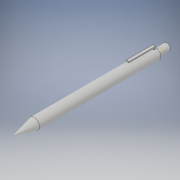
# Autodesk Inventor part: Pen
Saved by Autodesk Inventor 2017 (Build 210142000, 142)
## iProperties
Created: 2018-03-21
Part Number: Pen
Material: Generic
Document SubType Name: Modeling
Designer: landontracy
Density: 1 g/cm^3
Appearance: Default
Author: landontracy
Autodesk Inventor part; units mm, degrees
ref_plane "YZ Plane" through (0, 0, 0) normal (1, 0, 0) x (0, 1, 0)
sketch "Sketch1" plane through (0, 0, 0) normal (0, 0, 1) x (1, 0, 0)
  circle A0 centre (-3.4636, -0.3407) radius 4.445
  point P0 (0, 0)
  dimension "d0" = 8.89
  constraints: 1 centre point
  measures "d0" diameter of A0
extrude "Pen body" add sketch "Sketch1" along normal blind 101.6
ref_plane "Tip Plane" through (-3.4636, -0.3407, 119.38) normal (0, 0, 1) x (1, 0, 0)
sketch "Sketch2" plane through (-3.4636, -0.3407, 119.38) normal (0, 0, 1) x (1, 0, 0)
  circle A0 centre (0, 0) radius 0.0254
  point P0 (3.4636, 0.3407)
  dimension "d4" = 0.0508
  constraints: 1 centre point
  measures "d4" diameter of A0
loft "Body to Tip" add profiles "Sketch2" section 1 edges at (-7.9086, -0.3407, 101.6)
sketch "Sketch3" plane through (-3.4636, -0.3407, 0) normal (0, 0, -1) x (-1, 0, 0)
  point P0 (-3.4636, 0.3407)
sketch "Sketch4" plane through (-3.4636, -0.3407, 0) normal (0, 0, -1) x (-1, 0, 0)
  circle A0 centre (0, 0) radius 2.8396
  point P0 (-3.4636, 0.3407)
  constraints: 1 centre point
extrude "Click" add sketch "Sketch4" along normal blind 9.525
ref_plane "Clip" through (0, 4.0132, 0) normal (0, 1, 0) x (-1, 0, 0)
sketch "Clip extention" plane through (0, 4.0132, 0) normal (0, 1, 0) x (-1, 0, 0)
  point P0 (0, 0)
sketch "Clips extension's extension" plane through (0, 4.0132, 0) normal (0, 1, 0) x (-1, 0, 0)
  point P0 (0, 0)
sketch "Sketch7" plane through (0, 4.0132, 0) normal (0, 1, 0) x (-1, 0, 0)
  line L0 (4.5996, 1.2363) -> (2.3394, 1.2363)
  line L1 (2.3394, 1.2363) -> (2.3394, 2.4001)
  line L2 (2.3394, 2.4001) -> (4.5996, 2.4001)
  line L3 (4.5996, 2.4001) -> (4.5996, 1.2363)
  point P0 (0, 0)
  constraints: 8 end point, 2 parallel, 1 horizontal, 1 perpendicular
extrude "Extrusion3" add sketch "Sketch7" along normal blind 2.032
sketch "Sketch8" plane through (-4.5996, 4.0132, 2.4001) normal (0, 0, 1) x (1, 0, 0)
  line L0 (0, 0) -> (0, 2.032) projected
  line L1 (2.2602, 0) -> (2.2602, 2.032) projected
  line L2 (0, 2.032) -> (2.2602, 2.032)
  line L3 (2.2602, 2.032) -> (2.2602, 1.1849)
  line L4 (2.2602, 1.1849) -> (0, 1.1849)
  line L5 (0, 1.1849) -> (0, 2.032)
  point P0 (4.5996, -4.0132)
  constraints: 8 end point, 2 parallel, 1 horizontal, 1 perpendicular, 1 point on line
extrude "Extrusion4" add sketch "Sketch8" along normal blind 21.082
body "Solid1"
